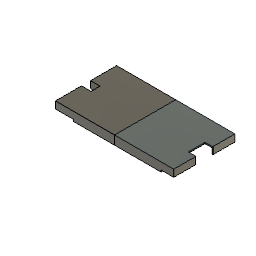
battery_cap (Autodesk Fusion 360 design; units mm, degrees)
part number: 2025-12-02-09-40-12-626
part number: 2025-12-02-11-55-00-746
Autodesk Fusion 360 part; units mm, degrees
sketch "Sketch1" plane through (0, 0, 0) normal (0, 0, 1) x (1, 0, 0)
  line L0 (0, 0) -> (464, 0)
  line L1 (464, 0) -> (464, 240)
  line L2 (464, 240) -> (0, 240)
  line L3 (0, 240) -> (0, 0)
  dimension "d1" = 464
  dimension "d2" = 240
  constraint horizontal L0
  constraint vertical L1
  constraint horizontal L2
  constraint vertical L3
  constraint coincident L0.start L3.end
  measures "d1" distance of L1 L3
  measures "d2" distance of L0 L2
extrude "Extrude1" add sketch "Sketch1" along normal blind 5 makes body 1
sketch "Sketch2" plane through (0, 0, 0) normal (0, 0, 1) x (1, 0, 0)
  line L0 (70, 240) -> (414, 240)
  line L1 (414, 240) -> (414, 220)
  line L2 (414, 220) -> (70, 220)
  line L3 (70, 220) -> (70, 240)
  line L4 (464, 0) -> (464, 240)
  line L5 (0, 240) -> (0, 0)
  dimension "d5" = 20
  dimension "d6" = 50
  dimension "d7" = 70
  constraint horizontal L0
  constraint vertical L1
  constraint horizontal L2
  constraint vertical L3
  measures "d5" distance of L0 L2
  measures "d6" distance of L1 L4
  measures "d7" distance of L3 L5
extrude "Extrude2" add sketch "Sketch2" against normal blind 30 separate body makes body 2
ref_plane "WorkPlane1" through (232, 120, 2.5) normal (0, -1, 0) x (1, 0, 0)
sketch "Sketch3" plane through (0, 0, -30) normal (0, 0, -1) x (1, 0, 0)
  line L0 (70, -20) -> (414, -20)
  line L1 (414, -20) -> (414, 0)
  line L2 (414, 0) -> (70, 0)
  line L3 (70, 0) -> (70, -20)
  line L4 (70, -224.25) -> (414, -224.25)
  line L5 (414, -224.25) -> (414, -229.25)
  line L6 (414, -229.25) -> (70, -229.25)
  line L7 (70, -229.25) -> (70, -224.25)
  line L8 (70, -240) -> (414, -240)
  dimension "d16" = 5
  dimension "d17" = 10.75
  constraint horizontal L4
  constraint vertical L5
  constraint horizontal L6
  constraint vertical L7
  measures "d16" distance of L4 L6
  measures "d17" distance of L6 L8
extrude "Extrude3" add sketch "Sketch3" along normal blind 5 contours L4 L5 L6 L7 bodies 2
mirror "Mirror2" about plane through (232, 120, 2.5) normal (0, -1, 0) of bodies 2 makes body 3
sketch "Sketch4" plane through (0, 0, 5) normal (0, 0, 1) x (-1, 0, 0)
  line L0 (0, -240) -> (0, 0)
  line L1 (0, 0) -> (-464, 0)
  line L2 (-464, 0) -> (-464, -240)
  line L3 (-464, -240) -> (0, -240)
  line L4 (-464, -87.5) -> (-434, -87.5)
  line L5 (-434, -87.5) -> (-434, -152.5)
  line L6 (-434, -152.5) -> (-464, -152.5)
  line L7 (-464, -152.5) -> (-464, -87.5)
  dimension "d18" = 30
  dimension "d19" = 65
  dimension "d20" = 87.5
  constraint horizontal L4
  constraint vertical L5
  constraint horizontal L6
  constraint vertical L7
  constraint coincident L2 L4.start
  measures "d18" distance of L5 L7
  measures "d19" distance of L4 L6
  measures "d20" distance of L3 L6
extrude "Extrude4" cut sketch "Sketch4" against normal blind 20 contours L2 L4 L5 L6 L7 bodies 1
fillet "Fillet1" radius 2.5 1 edges at (434, 152.5, 2.5) on bodies 1
fillet "Fillet1" radius 2.5 1 edges at (434, 87.5, 2.5) on bodies 1
fillet "Fillet1" radius 2.5 2 edges at (464, 152.5, 2.5) (464, 87.5, 2.5) on bodies 1
sketch "Sketch5" plane through (0, 0, 5) normal (0, 0, 1) x (-1, 0, 0)
  arc A0 (-464, -85) -> (-461.5, -87.5) centre (-461.5, -85) ccw
  line L0 (-461.5, -87.5) -> (-436.5, -87.5)
  arc A1 (-434, -90) -> (-436.5, -87.5) centre (-436.5, -90) ccw
  line L1 (-434, -90) -> (-434, -150)
  arc A2 (-436.5, -152.5) -> (-434, -150) centre (-436.5, -150) ccw
  line L2 (-436.5, -152.5) -> (-461.5, -152.5)
  arc A3 (-461.5, -152.5) -> (-464, -155) centre (-461.5, -155) ccw
  line L3 (-464, -155) -> (-464, -240)
  line L4 (-464, -240) -> (0, -240)
  line L5 (0, -240) -> (0, 0)
  line L6 (0, 0) -> (-464, 0)
  line L7 (-464, 0) -> (-464, -85)
  line L8 (-37.5, -102.5) -> (37.5, -102.5)
  line L9 (37.5, -102.5) -> (37.5, -137.5)
  line L10 (37.5, -137.5) -> (-37.5, -137.5)
  line L11 (-37.5, -137.5) -> (-37.5, -102.5)
  line L12 (-37.5, -102.5) -> (37.5, -137.5) construction
  line L13 (37.5, -102.5) -> (-37.5, -137.5) construction
  point P0 (0, -120)
  dimension "d29" = 35
  dimension "d30" = 75
  constraint horizontal L8
  constraint perpendicular L8 L9
  constraint parallel L8 L10
  constraint parallel L9 L11
  constraint coincident L12 P0
  constraint coincident L13 P0
  constraint midpoint L5 P0
  measures "d29" distance of L8 L10
  measures "d30" distance of L9 L11
extrude "Extrude5" cut sketch "Sketch5" against normal blind 20 contours L5 L8 L10 L11 bodies 1
ref_plane "WorkPlane2" through (232, 42.5, 2.5) normal (1, 0, 0) x (0, 1, 0)
sketch "Sketch6" plane through (0, 0, 0) normal (0, 0, -1) x (1, 0, 0)
  line L0 (37.5, -137.5) -> (0, -137.5)
  line L1 (0, -137.5) -> (0, -240)
  line L2 (0, -240) -> (464, -240)
  line L3 (464, -240) -> (464, -155)
  arc A0 (464, -155) -> (461.5, -152.5) centre (461.5, -155) ccw
  line L4 (461.5, -152.5) -> (436.5, -152.5)
  arc A1 (434, -150) -> (436.5, -152.5) centre (436.5, -150) ccw
  line L5 (434, -150) -> (434, -90)
  arc A2 (436.5, -87.5) -> (434, -90) centre (436.5, -90) ccw
  line L6 (436.5, -87.5) -> (461.5, -87.5)
  arc A3 (461.5, -87.5) -> (464, -85) centre (461.5, -85) ccw
  line L7 (464, -85) -> (464, 0)
  line L8 (464, 0) -> (0, 0)
  line L9 (0, 0) -> (0, -102.5)
  line L10 (0, -102.5) -> (37.5, -102.5)
  line L11 (37.5, -102.5) -> (37.5, -137.5)
  line L12 (69.692, -235.8943) -> (5, -235.8943)
  line L13 (5, -235.8943) -> (5, -142.4685)
  line L14 (5, -142.4685) -> (41.9514, -142.4685)
  line L15 (41.9514, -142.4685) -> (41.9514, -96.9772)
  line L16 (41.9514, -96.9772) -> (5, -96.9772)
  line L17 (5, -96.9772) -> (5, -5)
  line L18 (5, -5) -> (70, -5)
  constraint parallel L2 L12
  constraint perpendicular L12 L13
  constraint perpendicular L13 L14
  constraint perpendicular L0 L15
  constraint perpendicular L15 L16
  constraint perpendicular L8 L17
extrude "Extrude6" add sketch "Sketch6" along normal blind 23 thin wall 3 inside separate body makes body 4
combine "Combine1" operation add target body 4 tool bodies 3 2 1
split "Split1" by plane through (232, 42.5, 2.5) normal (1, 0, 0) bodies 4 makes body 5 at (299.3333, 130, 5)
sketch "Sketch7" plane through (0, 0, -23) normal (0, 0, -1) x (1, 0, 0)
  line L0 (414, -237) -> (414, -240)
  line L1 (414, -240) -> (464, -240)
  line L2 (464, -240) -> (464, -155)
  arc A0 (464, -155) -> (461.5, -152.5) centre (461.5, -155) ccw
  line L3 (461.5, -152.5) -> (436.5, -152.5)
  arc A1 (434, -150) -> (436.5, -152.5) centre (436.5, -150) ccw
  line L4 (434, -150) -> (434, -90)
  arc A2 (436.5, -87.5) -> (434, -90) centre (436.5, -90) ccw
  line L5 (436.5, -87.5) -> (461.5, -87.5)
  arc A3 (461.5, -87.5) -> (464, -85) centre (461.5, -85) ccw
  line L6 (464, -85) -> (464, 0)
  line L7 (464, 0) -> (414, 0)
  line L8 (414, 0) -> (414, -3)
  line L9 (414, -3) -> (461, -3)
  line L10 (461, -3) -> (461, -84.5)
  line L11 (461, -84.5) -> (436.5, -84.5)
  arc A4 (436.5, -84.5) -> (431, -90) centre (436.5, -90) ccw
  line L12 (431, -90) -> (431, -150)
  arc A5 (431, -150) -> (436.5, -155.5) centre (436.5, -150) ccw
  line L13 (436.5, -155.5) -> (461, -155.5)
  line L14 (461, -155.5) -> (461, -237)
  line L15 (461, -237) -> (414, -237)
  line L16 (461, -84.5) -> (461, -155.5)
  constraint coincident L10.end L11.start
  constraint coincident L13.end L14.start
extrude "Extrude7" cut sketch "Sketch7" against normal blind 23 contours L3 A1 L4 A2 L5 L11 A4 L12 A5 L13 L16 bodies 5
sketch "Sketch8" plane through (0, 0, 5) normal (0, 0, 1) x (-1, 0, 0)
  line L0 (-232, -240) -> (-232, 0)
  line L1 (-232, 0) -> (-464, 0)
  line L2 (-464, 0) -> (-464, -85)
  arc A0 (-464, -85) -> (-461.5, -87.5) centre (-461.5, -85) ccw
  line L3 (-461.5, -87.5) -> (-436.5, -87.5)
  arc A1 (-434, -90) -> (-436.5, -87.5) centre (-436.5, -90) ccw
  line L4 (-434, -90) -> (-434, -150)
  arc A2 (-436.5, -152.5) -> (-434, -150) centre (-436.5, -150) ccw
  line L5 (-436.5, -152.5) -> (-461.5, -152.5)
  arc A3 (-461.5, -152.5) -> (-464, -155) centre (-461.5, -155) ccw
  line L6 (-464, -155) -> (-464, -240)
  line L7 (-464, -240) -> (-232, -240)
component "body" placed x (1, 0, 0) y (0, 1, 0) z (0, 0, 1) at (0, 0, 0)
equation "d20 = 120 mm - ( 65 / 2 ) * 1 mm"
